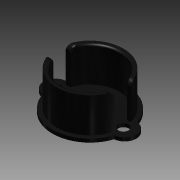
# Autodesk Inventor part: polulu_caster
Saved by Autodesk Inventor 2014 (Build 180170000, 170)
## iProperties
Created: 2015-05-04
Part Number: polulu_caster
Material: Generic
Document SubType Name: Modeling
Designer: Gabriel
Density: 1 g/cm^3
Appearance: Default
Author: Gabriel
Autodesk Inventor part; units mm, degrees
ref_plane "YZ Plane" through (0, 0, 0) normal (1, 0, 0) x (0, 1, 0)
ref_plane "XZ Plane" through (0, 0, 0) normal (0, 1, 0) x (-1, 0, 0)
ref_plane "XY Plane" through (0, 0, 0) normal (0, 0, 1) x (1, 0, 0)
sketch "Sketch1" plane through (0, 0, 0) normal (0, 1, 0) x (-1, 0, 0)
  circle A0 centre (-7.366, 0) radius 1.143
  circle A1 centre (7.366, 0) radius 1.143
  line L0 (10.16, 0) -> (10.16, 0)
  line L1 (10.16, 0) -> (10.16, 0)
  line L2 (-10.16, 0) -> (-10.16, 0)
  line L3 (-10.16, 0) -> (-10.16, 0)
  arc A2 (-10.16, 0) -> (-7.62, -2.54) centre (-7.62, 0) ccw
  arc A3 (-7.8454, 2.53) -> (-10.16, 0) centre (-7.62, 0) ccw
  arc A4 (10.16, 0) -> (7.8454, 2.53) centre (7.62, 0) ccw
  arc A5 (7.8454, -2.53) -> (10.16, 0) centre (7.62, 0) ccw
  arc A6 (7.8454, 2.53) -> (-7.8454, 2.53) centre (0, 0) ccw
  arc A7 (-7.8454, -2.53) -> (7.8454, -2.53) centre (0, 0) ccw
  dimension "d2" = 2.286
  dimension "d15" = 2.54
  dimension "d16" = 2.54
  dimension "d17" = 2.54
  constraints: 13 point on circle, 8 centre point, 8 end point, 4 tangent, 1 concentric
  measures "d2" diameter of A0
  measures "d15" radius of A2
  measures "d16" radius of A3
  measures "d17" radius of A4
extrude "Extrusion1" add sketch "Sketch1" along normal blind 0.762
sketch "Sketch2" plane through (0, 0.762, 0) normal (0, 1, 0) x (1, 0, 0)
  point P0 (0, 0)
sketch "Sketch3" plane through (0, 0.762, 0) normal (0, 1, 0) x (1, 0, 0)
  line L0 (-7.2575, -1.2599) -> (-7.2559, -1.2599)
  line L1 (-7.2559, -1.2599) -> (-7.2559, -1.269)
  line L2 (-7.1482, -1.778) -> (-6.096, -1.778)
  line L3 (-7.2559, 1.269) -> (-7.2559, 1.27)
  line L4 (-7.1482, 1.778) -> (-6.096, 1.778)
  arc A0 (7.1482, 1.778) -> (-7.1482, 1.778) centre (0, 0) ccw
  arc A1 (-7.2557, 1.27) -> (-7.2559, 1.269) centre (0, 0) ccw
  arc A2 (-7.2575, -1.2599) -> (-7.2559, -1.269) centre (0, 0) ccw
  arc A3 (-7.1482, -1.778) -> (7.1482, -1.778) centre (0, 0) ccw
  line L5 (-7.2575, -1.2599) -> (-7.2559, -1.2599)
  line L6 (6.096, -1.778) -> (7.1482, -1.778)
  line L7 (6.096, 1.778) -> (7.1482, 1.778)
  arc A4 (6.096, 1.778) -> (-6.096, 1.778) centre (0, 0) ccw
  arc A5 (-6.096, -1.778) -> (6.096, -1.778) centre (0, 0) ccw
  constraints: 16 end point, 13 point on circle, 6 centre point, 4 perpendicular, 2 coincident, 1 parallel
extrude "Extrusion2" add sketch "Sketch3" along normal blind 7.62 contours A0 L7 A4 L4 | L2 A5 L6 A1
fillet "Fillet1" radius 1.27 4 edges at (6.6221, 8.382, 1.778) (-6.6221, 8.382, 1.778) (-6.6221, 8.382, -1.778) (6.6221, 8.382, -1.778)
fillet "Fillet2" radius 0.508 10 edges at (5.9835, 7.9854, -2.126) (6.096, 3.937, -1.778) (-5.9838, 7.9847, -2.1254) (-6.096, 3.937, -1.778) (0, 8.382, -6.35) (-5.9835, 7.9854, 2.126) (-6.096, 3.937, 1.778) (5.9835, 7.9854, 2.126) (6.096, 3.937, 1.778) (0, 8.382, 6.35)
body "Solid1"
